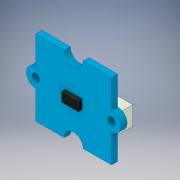
# Autodesk Inventor part: GROVE-VL53L0X
Saved by Autodesk Inventor 2019 (Build 230136000, 136)
## iProperties
Created: 2019-10-03
Part Number: GROVE-VL53L0X
Material: Plastique ABS
Document SubType Name: Modeling
Designer: Sébastien DI MERCURIO
Density: 1.06 g/cm^3
Appearance: Bleu ciel moyen
Mass: 0.667744 g
Surface Area: 9.53805 cm^2
Volume: 0.629947 cm^3
Author: Sébastien DI MERCURIO
Autodesk Inventor part; units mm, degrees
ref_plane "YZ Plane" through (0, 0, 0) normal (1, 0, 0) x (0, 1, 0)
ref_plane "XZ Plane" through (0, 0, 0) normal (0, 1, 0) x (-1, 0, 0)
ref_plane "XY Plane" through (0, 0, 0) normal (0, 0, 1) x (1, 0, 0)
sketch "Esquisse1" plane through (0, 0, 0) normal (0, 0, 1) x (1, 0, 0)
  point P0 (0, 0)
sketch "Esquisse2" plane through (0, 0, 0) normal (0, 0, 1) x (1, 0, 0)
  line L0 (-10, 10) -> (10, 10)
  line L1 (10, 10) -> (10, -10)
  line L2 (10, -10) -> (-10, -10)
  line L3 (-10, -10) -> (-10, 10)
  point P0 (0, 0)
  dimension "d0" = 20
  dimension "d1" = 10
  dimension "d2" = 10
  constraints: 8 end point, 2 parallel, 2 perpendicular, 1 horizontal
  measures "d0" distance of L0.start L0.end
  measures "d1" horizontal distance of point (0, 0) L0.start
  measures "d2" horizontal distance of point (0, 0) L0.start
extrude "Extrusion1" add sketch "Esquisse2" along normal blind 1.6
sketch "Esquisse3" plane through (0, 0, 1.6) normal (0, 0, 1) x (1, 0, 0)
  line L0 (-10, 10) -> (-10, -10) projected
  circle A0 centre (-10, 0) radius 2.5
  line L1 (10, -10) -> (10, 10) projected
  circle A1 centre (10, 0) radius 2.5
  point P0 (0, 0)
  dimension "d5" = 5
  constraints: 2 centre point, 2 midpoint, 1 equal radius
  measures "d5" diameter of A0
extrude "Extrusion2" add sketch "Esquisse3" against normal blind 1.6
sketch "Esquisse4" plane through (0, 0, 1.6) normal (0, 0, 1) x (1, 0, 0)
  circle A0 centre (10, 0) radius 1
  circle A1 centre (-10, 0) radius 1
  line L0 (10, -10) -> (-10, -10) projected
  circle A2 centre (0, -10) radius 2.5
  circle A3 centre (0, 10) radius 2.5
  line L1 (10, 0) -> (0, 0)
  line L2 (0, 0) -> (-10, 0)
  line L3 (0, -10) -> (0, 0)
  line L4 (0, 0) -> (0, 10)
  line L5 (-10, 10) -> (10, 10) projected
  dimension "d8" = 5
  dimension "d9" = 2
  constraints: 8 end point, 4 centre point, 3 equal length, 2 equal radius, 1 collinear, 1 horizontal, 1 midpoint, 1 perpendicular, 1 vertical
  measures "d8" diameter of A2
  measures "d9" diameter of A0
extrude "Extrusion3" cut sketch "Esquisse4" against normal through all
sketch "Esquisse5" plane through (0, 0, 1.6) normal (0, 0, 1) x (1, 0, 0)
  line L0 (2.25, -1.25) -> (-2.25, -1.25)
  line L1 (-2.25, -1.25) -> (-2.25, 1.25)
  line L2 (-2.25, 1.25) -> (2.25, 1.25)
  line L3 (2.25, 1.25) -> (2.25, -1.25)
  line L4 (-10, -10) -> (-2.5, -10) projected
  line L5 (-2.5, 10) -> (-10, 10) projected
  arc A0 (2.5, -10) -> (-2.5, -10) centre (0, -10) ccw projected
  line L6 (-10, -2.5) -> (-10, -10) projected
  line L7 (-10, -10) -> (-10, 10) construction
  line L8 (10, 2.5) -> (10, 10) construction
  line L9 (10, -10) -> (10, 10) construction
  line L10 (2.25, -1.25) -> (10, -1.25) construction
  line L11 (-2.25, -1.25) -> (-10, -1.25) construction
  line L12 (10, -10) -> (-10, -10) construction
  line L13 (10, 10) -> (-10, 10) construction
  line L14 (2.25, 1.25) -> (2.25, 10) construction
  line L15 (2.25, -1.25) -> (2.25, -10) construction
  point P0 (0, 0)
  dimension "d12" = 4.5
  dimension "d13" = 2.5
  constraints: 24 end point, 6 collinear, 5 point on line, 4 perpendicular, 2 parallel, 1 horizontal
  measures "d12" distance of L0.start L0.end
  measures "d13" distance of L2.end L0.start
extrude "Extrusion4" add sketch "Esquisse5" along normal blind 1
sketch "Esquisse6" plane through (0, 0, 0) normal (0, 0, -1) x (-1, 0, 0)
  line L0 (6, -8) -> (-6, -8)
  line L1 (-6, -8) -> (-6, -3)
  line L2 (-6, -3) -> (6, -3)
  line L3 (6, -3) -> (6, -8)
  line L4 (2.5, -10) -> (10, -10) projected
  line L5 (2.5, 10) -> (10, 10) construction
  line L6 (10, -10) -> (10, 10) construction
  line L7 (-2.5, -10) -> (-10, -10) construction
  line L8 (-10, 2.5) -> (-10, 10) construction
  line L9 (-10, -10) -> (-10, 10) construction
  line L10 (6, -3) -> (10, -3) construction
  line L11 (10, -2.5) -> (10, -10) construction
  line L12 (-6, -3) -> (-10, -3) construction
  point P0 (0, 0)
  dimension "d16" = 12
  dimension "d17" = 5
  dimension "d18" = 2
  constraints: 16 end point, 3 point on line, 2 parallel, 2 perpendicular, 2 vertical, 1 collinear, 1 horizontal
  measures "d16" distance of L0.start L0.end
  measures "d17" distance of L2.end L0.start
  measures "d18" distance between parallel lines of L0 L4
extrude "Extrusion5" add sketch "Esquisse6" along normal blind 8
sketch "Esquisse7" plane through (0, 0, -8) normal (0, 0, -1) x (-1, 0, 0)
  line L0 (5.2, -7.2) -> (-5.2, -7.2)
  line L1 (-5.2, -7.2) -> (-5.2, -3.8)
  line L2 (-5.2, -3.8) -> (5.2, -3.8)
  line L3 (5.2, -3.8) -> (5.2, -7.2)
  line L4 (-6, -8) -> (6, -8) projected
  line L5 (6, -3) -> (-6, -3) projected
  line L6 (6, -8) -> (6, -3) projected
  line L7 (-6, -3) -> (-6, -8) projected
  point P0 (0, 0)
  dimension "d21" = 0.8
  dimension "d22" = 0.8
  dimension "d23" = 0.8
  dimension "d24" = 0.8
  constraints: 8 end point, 2 parallel, 1 horizontal, 1 perpendicular
  measures "d21" distance between parallel lines of L0 L4
  measures "d22" distance between parallel lines of L5 L2
  measures "d23" distance between parallel lines of L3 L6
  measures "d24" distance between parallel lines of L7 L1
extrude "Extrusion6" cut sketch "Esquisse7" against normal blind 7 contours L0 L1 L2 L3
equation "\"d1\" = 0.5 * d0"
equation "\"d2\" = d1"
equation "\"d22\" = d21"
equation "\"d23\" = d22"
equation "\"d24\" = d22"
